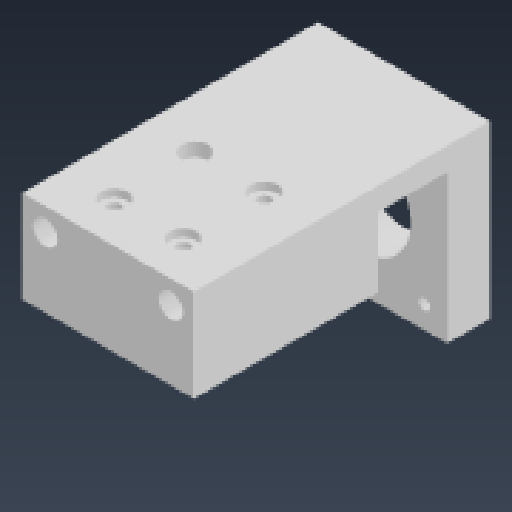
# Autodesk Inventor part: PRINTED z motor mount right
Saved by Autodesk Inventor 2024.3 (Build 283343000, 343)
## iProperties
Created: 2024-07-29
Part Number: PRINTED z motor mount right
Material: Generic
Document SubType Name: Modeling
Designer: mateu
Density: 1 g/cm^3
Appearance: Default
Author: mateu
Autodesk Inventor part; units mm, degrees
ref_plane "YZ Plane" through (0, 0, 0) normal (1, 0, 0) x (0, 1, 0)
ref_plane "XZ Plane" through (0, 0, 0) normal (0, 1, 0) x (-1, 0, 0)
ref_plane "XY Plane" through (0, 0, 0) normal (0, 0, 1) x (1, 0, 0)
sketch "Sketch1" plane through (0, 0, 0) normal (0, 0, 1) x (1, 0, 0)
  line L0 (21.025, -17.1393) -> (17.0778, -21.075) projected
  line L1 (21.075, 17.0778) -> (21.025, -17.1393) projected
  line L2 (17.1393, 21.025) -> (21.075, 17.0778) projected
  line L3 (-17.0778, 21.075) -> (17.1393, 21.025) projected
  line L4 (-21.025, 17.1393) -> (-17.0778, 21.075) projected
  line L5 (-21.075, -17.0778) -> (-21.025, 17.1393) projected
  line L6 (-17.1393, -21.025) -> (-21.075, -17.0778) projected
  line L7 (17.0778, -21.075) -> (-17.1393, -21.025) projected
  circle A0 centre (-15.5226, -15.4774) radius 1.3645 projected
  circle A1 centre (15.5226, 15.4774) radius 1.3645 projected
  circle A2 centre (0, 0) radius 11.1 projected
  circle A3 centre (-15.4774, 15.5226) radius 1.3645 projected
  circle A4 centre (15.4774, -15.5226) radius 1.3645 projected
  circle A5 centre (0, 0) radius 12.1
  line L8 (21.075, 17.0778) -> (17.1393, 17.0778)
  line L9 (17.1393, 17.0778) -> (17.1393, 21.025)
  line L10 (17.1393, 21.025) -> (21.075, 21.025)
  line L11 (21.075, 21.025) -> (21.075, 17.0778)
  line L12 (-17.1393, -21.025) -> (-21.075, -21.025)
  line L13 (-21.075, -21.025) -> (-21.075, -17.0778)
  line L14 (-21.075, -17.0778) -> (-17.1393, -17.0778)
  line L15 (-17.1393, -17.0778) -> (-17.1393, -21.025)
  line L16 (-17.1394, -21.125) -> (17.0777, -21.175) projected
  line L17 (-21.125, 17.1394) -> (-21.175, -17.0777) projected
  line L18 (21.125, -17.1394) -> (21.175, 17.0777) projected
  line L19 (17.1394, 21.125) -> (-17.0777, 21.175) projected
  line L20 (17.1394, 21.125) -> (21.175, 21.125)
  line L21 (21.175, 21.125) -> (21.175, 17.0777)
  line L22 (21.175, 17.0777) -> (17.1394, 17.0777)
  line L23 (17.1394, 17.0777) -> (17.1394, 21.125)
  line L24 (-17.1394, -21.125) -> (-21.175, -21.125)
  line L25 (-21.175, -21.125) -> (-21.175, -17.0777)
  line L26 (-21.175, -17.0777) -> (-17.1394, -17.0777)
  line L27 (-17.1394, -17.0777) -> (-17.1394, -21.125)
  line L28 (-21.175, -21.125) -> (21.175, -21.125)
  line L29 (21.175, -21.125) -> (21.175, 21.125)
  line L30 (21.175, 21.125) -> (-21.175, 21.125)
  line L31 (-21.175, 21.125) -> (-21.175, -21.125)
  point P0 (0, 0)
  dimension "d0" = 1
  constraints: 40 end point, 10 parallel, 5 horizontal, 5 perpendicular, 1 centre point
  measures "d0" radial gap between concentric circles of A2 A5
extrude "Extrusion1" add sketch "Sketch1" along normal blind 7.5 contours L1 L22 L29 L28 L27 L7 L0 | L0 L7 L15 L14 L5 L4 L3 L9 L8 L1 | L8 L9 L2 | L2 L10 L11 | L11 L10 L23 L20 L21 L22 | L12 L13 L6 | L27 L24 L25 L26 L13 L12 | L6 L14 L15 | L3 L4 L5 L26 L31 L30 L23
sketch "Sketch2" plane through (0, 0, 7.5) normal (0, 0, 1) x (1, 0, 0)
  arc A0 (-1.3547, 7.0848) -> (-1.824, -6.9788) centre (0, 0) ccw
  line L0 (-1.824, -6.9788) -> (52.9102, -21.2846)
  arc A1 (52.9102, -21.2846) -> (54.2116, 17.7095) centre (57.9677, -1.9346) ccw
  line L1 (54.2116, 17.7095) -> (-1.3547, 7.0848)
  line L2 (1.9235, 5.7586) -> (49.8414, 14.9208)
  arc A2 (50.6727, 15.052) -> (49.8414, 14.9208) centre (50.2992, 14.7197) ccw
  line L3 (50.6727, 15.052) -> (50.6801, 15.0435)
  spline S0 degree 3 poles (50.6801, 15.0435) (50.7219, 14.9959) (50.7686, 14.9492) (50.8593, 14.8771) (50.9053, 14.847) (50.9855, 14.8139) (51.0188, 14.8048) (51.0975, 14.7994) (51.1299, 14.8087) (51.1978, 14.8319) (51.2575, 14.8594) (51.2738, 14.8659) knots 0 0 0 0 0.221578 0.221578 0.405224 0.405224 0.524808 0.524808 0.681199 0.681199 1 1 1 1
  spline S1 degree 3 poles (51.2738, 14.8659) (51.3213, 14.8848) (51.3717, 14.8983) (51.4381, 14.9355) (51.4654, 14.9544) (51.5177, 15.0213) (51.536, 15.06) (51.5803, 15.1932) (51.5866, 15.3045) (51.5828, 15.4032) knots 0 0 0 0 0.321396 0.321396 0.48066 0.48066 0.635294 0.635294 1 1 1 1
  line L4 (51.5828, 15.4032) -> (51.5823, 15.4144)
  arc A3 (52.4883, 15.7215) -> (51.5823, 15.4144) centre (52.082, 15.43) ccw
  ellipse E0 centre (52.6181, 16.5825) end of major axis (52.9222, 15.4382) minor radius 0.4695 (52.4883, 15.7215) -> (52.7342, 15.4739) ccw
  line L5 (52.7342, 15.4739) -> (53.3062, 15.5833)
  spline S2 degree 3 poles (53.3062, 15.5833) (53.3285, 15.6089) (53.3465, 15.6383) (53.3759, 15.7001) (53.3876, 15.7332) (53.4154, 15.8335) (53.4254, 15.9062) (53.43, 15.9756) knots 0 0 0 0 0.246113 0.246113 0.495831 0.495831 1 1 1 1
  line L6 (53.43, 15.9756) -> (53.4307, 15.9869)
  arc A4 (54.3639, 16.1976) -> (53.4307, 15.9869) centre (53.9294, 15.9501) ccw
  line L7 (54.3639, 16.1976) -> (54.3693, 16.1877)
  spline S3 degree 3 poles (54.3693, 16.1877) (54.4048, 16.1244) (54.4473, 16.0602) (54.5277, 15.9698) (54.5647, 15.9356) (54.6338, 15.8924) (54.664, 15.8787) (54.7363, 15.8619) (54.7701, 15.8644) (54.8153, 15.8718) knots 0 0 0 0 0.371919 0.371919 0.619946 0.619946 0.788977 0.788977 1 1 1 1
  line L8 (54.8153, 15.8718) -> (54.9027, 15.8885)
  spline S4 degree 3 poles (54.9027, 15.8885) (54.9046, 15.8889) (54.9067, 15.8893) (54.91, 15.89) (54.9117, 15.8903) (54.9132, 15.8905) knots 0 0 0 0 0.573872 0.573872 1 1 1 1
  line L9 (54.9132, 15.8905) -> (55.0804, 15.9225)
  spline S5 degree 3 poles (55.0804, 15.9225) (55.0932, 15.9274) (55.1129, 15.936) (55.1525, 15.9644) (55.1681, 15.9786) (55.2105, 16.0255) (55.2333, 16.0625) (55.2889, 16.1774) (55.3125, 16.2676) (55.327, 16.3518) knots 0 0 0 0 0.157005 0.157005 0.276336 0.276336 0.51523 0.51523 1 1 1 1
  line L10 (55.327, 16.3518) -> (55.3289, 16.3629)
  arc A5 (56.2789, 16.4749) -> (55.3289, 16.3629) centre (55.821, 16.2743) ccw
  ellipse E1 centre (56.5798, 17.2686) end of major axis (56.6442, 16.1081) minor radius 0.4625 (56.2789, 16.4749) -> (56.4624, 16.1868) ccw
  line L11 (56.4624, 16.1868) -> (57.173, 16.3227)
  ellipse E2 centre (56.96, 17.031) end of major axis (56.9523, 16.1396) minor radius 0.3594 (57.173, 16.3227) -> (57.2529, 16.5276) ccw
  line L12 (57.2529, 16.5276) -> (57.256, 16.5385)
  arc A6 (58.2125, 16.5506) -> (57.256, 16.5385) centre (57.7361, 16.3989) ccw
  line L13 (58.2125, 16.5506) -> (58.2158, 16.5398)
  ellipse E3 centre (58.3562, 16.7592) end of major axis (58.4541, 16.2126) minor radius 0.1884 (58.2158, 16.5398) -> (58.2211, 16.5231) ccw
  line L14 (58.2211, 16.5231) -> (59.3878, 16.7461)
  arc A7 (60.1434, 16.4238) -> (59.3878, 16.7461) centre (59.6537, 16.3227) ccw
  line L15 (60.1434, 16.4238) -> (60.1456, 16.4127)
  spline S6 degree 3 poles (60.1456, 16.4127) (60.1579, 16.3506) (60.175, 16.2867) (60.2175, 16.1789) (60.2423, 16.1299) (60.2952, 16.0611) (60.3195, 16.0366) (60.385, 15.9926) (60.4177, 15.9844) (60.4881, 15.9705) (60.5536, 15.9645) (60.5709, 15.962) knots 0 0 0 0 0.221578 0.221578 0.405224 0.405224 0.524808 0.524808 0.681199 0.681199 1 1 1 1
  spline S7 degree 3 poles (60.5709, 15.962) (60.6214, 15.9546) (60.6719, 15.9411) (60.7479, 15.9402) (60.7811, 15.9429) (60.8598, 15.9747) (60.895, 15.999) (61, 16.0922) (61.0611, 16.1855) (61.1071, 16.2728) knots 0 0 0 0 0.321396 0.321396 0.48066 0.48066 0.635294 0.635294 1 1 1 1
  line L16 (61.1071, 16.2728) -> (61.1123, 16.2828)
  arc A8 (62.0505, 16.0958) -> (61.1123, 16.2828) centre (61.5529, 16.0464) ccw
  line L17 (62.0505, 16.0958) -> (62.0514, 16.0845)
  spline S8 degree 3 poles (62.0514, 16.0845) (62.0572, 16.0215) (62.0676, 15.9562) (62.0985, 15.8445) (62.1181, 15.7932) (62.1635, 15.7193) (62.1851, 15.6924) (62.2456, 15.6417) (62.2773, 15.6302) (62.3459, 15.609) (62.4104, 15.5962) (62.4274, 15.5919) knots 0 0 0 0 0.221578 0.221578 0.405224 0.405224 0.524808 0.524808 0.681199 0.681199 1 1 1 1
  spline S9 degree 3 poles (62.4274, 15.5919) (62.4768, 15.5792) (62.5256, 15.5605) (62.6011, 15.5516) (62.6344, 15.5509) (62.716, 15.5743) (62.7536, 15.5948) (62.8677, 15.6765) (62.9382, 15.7629) (62.9931, 15.8449) knots 0 0 0 0 0.321396 0.321396 0.48066 0.48066 0.635294 0.635294 1 1 1 1
  line L18 (62.9931, 15.8449) -> (62.9993, 15.8543)
  arc A9 (63.9128, 15.5702) -> (62.9993, 15.8543) centre (63.4128, 15.5732) ccw
  line L19 (63.9128, 15.5702) -> (63.9126, 15.5589)
  spline S10 degree 3 poles (63.9126, 15.5589) (63.9118, 15.4956) (63.9152, 15.4296) (63.9343, 15.3154) (63.9484, 15.2622) (63.9858, 15.184) (64.0045, 15.155) (64.0594, 15.0982) (64.0897, 15.0835) (64.1557, 15.0553) (64.2185, 15.0358) (64.235, 15.0297) knots 0 0 0 0 0.221578 0.221578 0.405224 0.405224 0.524808 0.524808 0.681199 0.681199 1 1 1 1
  spline S11 degree 3 poles (64.235, 15.0297) (64.2828, 15.012) (64.3294, 14.9883) (64.4035, 14.9715) (64.4366, 14.9673) (64.5201, 14.982) (64.5597, 14.9985) (64.6817, 15.0679) (64.7608, 15.1464) (64.824, 15.2222) knots 0 0 0 0 0.321396 0.321396 0.48066 0.48066 0.635294 0.635294 1 1 1 1
  line L20 (64.824, 15.2222) -> (64.8312, 15.2309)
  arc A10 (65.71, 14.8529) -> (64.8312, 15.2309) centre (65.213, 14.9081) ccw
  line L21 (65.71, 14.8529) -> (65.7086, 14.8417)
  spline S12 degree 3 poles (65.7086, 14.8417) (65.7012, 14.7788) (65.6977, 14.7128) (65.7048, 14.5972) (65.7132, 14.5428) (65.7423, 14.4611) (65.7578, 14.4303) (65.8065, 14.3682) (65.8351, 14.3503) (65.8977, 14.3154) (65.9581, 14.2894) (65.9739, 14.2817) knots 0 0 0 0 0.221578 0.221578 0.405224 0.405224 0.524808 0.524808 0.681199 0.681199 1 1 1 1
  spline S13 degree 3 poles (65.9739, 14.2817) (66.0196, 14.259) (66.0634, 14.2306) (66.1355, 14.2062) (66.1679, 14.1985) (66.2525, 14.2044) (66.2935, 14.2167) (66.4222, 14.2729) (66.5091, 14.3428) (66.5798, 14.4116) knots 0 0 0 0 0.321396 0.321396 0.48066 0.48066 0.635294 0.635294 1 1 1 1
  line L22 (66.5798, 14.4116) -> (66.5879, 14.4195)
  arc A11 (67.4223, 13.9517) -> (66.5879, 14.4195) centre (66.9339, 14.0585) ccw
  line L23 (67.4223, 13.9517) -> (67.4198, 13.9407)
  spline S14 degree 3 poles (67.4198, 13.9407) (67.4058, 13.8789) (67.3955, 13.8136) (67.3904, 13.6979) (67.3932, 13.643) (67.4135, 13.5587) (67.4257, 13.5264) (67.4676, 13.4595) (67.4942, 13.4388) (67.5529, 13.3974) (67.6102, 13.3653) (67.6251, 13.356) knots 0 0 0 0 0.221578 0.221578 0.405224 0.405224 0.524808 0.524808 0.681199 0.681199 1 1 1 1
  spline S15 degree 3 poles (67.6251, 13.356) (67.6682, 13.3287) (67.7088, 13.2958) (67.7779, 13.264) (67.8093, 13.253) (67.8941, 13.25) (67.9362, 13.2579) (68.07, 13.3004) (68.1637, 13.3608) (68.2413, 13.4218) knots 0 0 0 0 0.321396 0.321396 0.48066 0.48066 0.635294 0.635294 1 1 1 1
  line L24 (68.2413, 13.4218) -> (68.2501, 13.4288)
  arc A12 (69.0311, 12.8764) -> (68.2501, 13.4288) centre (68.5565, 13.0337) ccw
  line L25 (69.0311, 12.8764) -> (69.0274, 12.8657)
  spline S16 degree 3 poles (69.0274, 12.8657) (69.0071, 12.8057) (68.99, 12.7419) (68.9729, 12.6273) (68.9698, 12.5724) (68.9812, 12.4864) (68.9901, 12.4531) (69.0247, 12.3822) (69.049, 12.3588) (69.103, 12.3115) (69.1567, 12.2736) (69.1705, 12.2627) knots 0 0 0 0 0.221578 0.221578 0.405224 0.405224 0.524808 0.524808 0.681199 0.681199 1 1 1 1
  spline S17 degree 3 poles (69.1705, 12.2627) (69.2105, 12.2311) (69.2475, 12.1941) (69.3128, 12.1553) (69.3429, 12.1411) (69.427, 12.1293) (69.4696, 12.1327) (69.6072, 12.161) (69.7067, 12.2112) (69.7902, 12.2638) knots 0 0 0 0 0.321396 0.321396 0.48066 0.48066 0.635294 0.635294 1 1 1 1
  line L26 (69.7902, 12.2638) -> (69.7997, 12.2699)
  arc A13 (70.5187, 11.6388) -> (69.7997, 12.2699) centre (70.0631, 11.8448) ccw
  line L27 (70.5187, 11.6388) -> (70.5139, 11.6285)
  spline S18 degree 3 poles (70.5139, 11.6285) (70.4874, 11.571) (70.4637, 11.5093) (70.4347, 11.3972) (70.426, 11.3429) (70.4283, 11.2562) (70.4336, 11.2221) (70.4607, 11.148) (70.4824, 11.1221) (70.5311, 11.0695) (70.5806, 11.0262) (70.5932, 11.0139) knots 0 0 0 0 0.221578 0.221578 0.405224 0.405224 0.524808 0.524808 0.681199 0.681199 1 1 1 1
  spline S19 degree 3 poles (70.5932, 11.0139) (70.6297, 10.9783) (70.6625, 10.9377) (70.7235, 10.8922) (70.7519, 10.8749) (70.8343, 10.8544) (70.8771, 10.8533) (71.0168, 10.8671) (71.121, 10.9067) (71.2096, 10.9502) knots 0 0 0 0 0.321396 0.321396 0.48066 0.48066 0.635294 0.635294 1 1 1 1
  line L28 (71.2096, 10.9502) -> (71.2197, 10.9553)
  arc A14 (71.8687, 10.2525) -> (71.2197, 10.9553) centre (71.4372, 10.5051) ccw
  line L29 (71.8687, 10.2525) -> (71.8629, 10.2428)
  spline S20 degree 3 poles (71.8629, 10.2428) (71.8305, 10.1884) (71.8005, 10.1295) (71.76, 10.021) (71.7456, 9.9679) (71.7389, 9.8815) (71.7406, 9.847) (71.7597, 9.7704) (71.7786, 9.7425) (71.8216, 9.6851) (71.8663, 9.6368) (71.8775, 9.6233) knots 0 0 0 0 0.221578 0.221578 0.405224 0.405224 0.524808 0.524808 0.681199 0.681199 1 1 1 1
  spline S21 degree 3 poles (71.8775, 9.6233) (71.9101, 9.584) (71.9385, 9.5402) (71.9944, 9.4886) (72.0209, 9.4684) (72.1006, 9.4394) (72.1431, 9.4339) (72.2835, 9.433) (72.3913, 9.4614) (72.4839, 9.4955) knots 0 0 0 0 0.321396 0.321396 0.48066 0.48066 0.635294 0.635294 1 1 1 1
  line L30 (72.4839, 9.4955) -> (72.4945, 9.4994)
  arc A15 (73.0665, 8.7327) -> (72.4945, 9.4994) centre (72.6637, 9.029) ccw
  line L31 (73.0665, 8.7327) -> (73.0597, 8.7237)
  spline S22 degree 3 poles (73.0597, 8.7237) (73.0218, 8.6729) (72.9858, 8.6175) (72.9341, 8.5138) (72.9143, 8.4625) (72.8986, 8.3773) (72.8966, 8.3428) (72.9077, 8.2646) (72.9235, 8.2349) (72.9603, 8.1733) (72.9997, 8.1206) (73.0094, 8.106) knots 0 0 0 0 0.221578 0.221578 0.405224 0.405224 0.524808 0.524808 0.681199 0.681199 1 1 1 1
  spline S23 degree 3 poles (73.0094, 8.106) (73.0377, 8.0635) (73.0614, 8.017) (73.1116, 7.9598) (73.1358, 7.937) (73.2121, 7.8998) (73.2537, 7.8899) (73.3933, 7.8743) (73.5035, 7.8913) (73.5991, 7.9155) knots 0 0 0 0 0.321396 0.321396 0.48066 0.48066 0.635294 0.635294 1 1 1 1
  line L32 (73.5991, 7.9155) -> (73.6101, 7.9184)
  arc A16 (74.0988, 7.096) -> (73.6101, 7.9184) centre (73.7292, 7.4328) ccw
  line L33 (74.0988, 7.096) -> (74.0911, 7.0877)
  spline S24 degree 3 poles (74.0911, 7.0877) (74.0538, 7.0474) (74.0178, 7.0036) (73.9564, 6.9135) (73.9287, 6.8641) (73.899, 6.7792) (73.8911, 6.7436) (73.8895, 6.6778) (73.8937, 6.6486) (73.9222, 6.5681) (73.9723, 6.4867) (74.0009, 6.4323) knots 0 0 0 0 0.238639 0.238639 0.473417 0.473417 0.629303 0.629303 0.759091 0.759091 1 1 1 1
  spline S25 degree 3 poles (74.0009, 6.4323) (74.0244, 6.387) (74.043, 6.3382) (74.0868, 6.276) (74.1084, 6.2507) (74.1802, 6.2055) (74.2206, 6.1912) (74.3576, 6.1607) (74.469, 6.1658) (74.5667, 6.1796) knots 0 0 0 0 0.321396 0.321396 0.48066 0.48066 0.635294 0.635294 1 1 1 1
  line L34 (74.5667, 6.1796) -> (74.5779, 6.1812)
  arc A17 (74.9755, 5.3111) -> (74.5779, 6.1812) centre (74.6442, 5.6856) ccw
  line L35 (74.9755, 5.3111) -> (74.9669, 5.3037)
  spline S26 degree 3 poles (74.9669, 5.3037) (74.9192, 5.2621) (74.8723, 5.2155) (74.7999, 5.125) (74.7697, 5.0791) (74.7364, 4.999) (74.7273, 4.9658) (74.7216, 4.887) (74.7308, 4.8546) (74.7538, 4.7866) (74.7812, 4.7269) (74.7876, 4.7105) knots 0 0 0 0 0.221578 0.221578 0.405224 0.405224 0.524808 0.524808 0.681199 0.681199 1 1 1 1
  spline S27 degree 3 poles (74.7876, 4.7105) (74.8063, 4.663) (74.8197, 4.6126) (74.8567, 4.5461) (74.8756, 4.5187) (74.9423, 4.4662) (74.9809, 4.4478) (75.114, 4.4031) (75.2253, 4.3965) (75.3239, 4.4) knots 0 0 0 0 0.321396 0.321396 0.48066 0.48066 0.635294 0.635294 1 1 1 1
  line L36 (75.3239, 4.4) -> (75.3352, 4.4005)
  arc A18 (75.6397, 3.4936) -> (75.3352, 4.4005) centre (75.3494, 3.9007) ccw
  line L37 (75.6397, 3.4936) -> (75.6304, 3.4872)
  spline S28 degree 3 poles (75.6304, 3.4872) (75.5786, 3.4508) (75.5271, 3.4093) (75.4457, 3.3269) (75.4108, 3.2844) (75.3693, 3.2083) (75.3567, 3.1761) (75.3429, 3.0984) (75.3487, 3.0652) (75.3644, 2.9952) (75.3854, 2.9329) (75.3901, 2.916) knots 0 0 0 0 0.221578 0.221578 0.405224 0.405224 0.524808 0.524808 0.681199 0.681199 1 1 1 1
  spline S29 degree 3 poles (75.3901, 2.916) (75.4037, 2.8668) (75.4118, 2.8152) (75.4416, 2.7452) (75.4575, 2.716) (75.5184, 2.6569) (75.5549, 2.6344) (75.6826, 2.5761) (75.7926, 2.5579) (75.891, 2.5511) knots 0 0 0 0 0.321396 0.321396 0.48066 0.48066 0.635294 0.635294 1 1 1 1
  line L38 (75.891, 2.5511) -> (75.9023, 2.5504)
  arc A19 (76.1103, 1.6167) -> (75.9023, 2.5504) centre (75.8641, 2.0518) ccw
  line L39 (76.1103, 1.6167) -> (76.1004, 1.6112)
  spline S30 degree 3 poles (76.1004, 1.6112) (76.045, 1.5804) (75.9895, 1.5446) (75.8999, 1.4711) (75.8608, 1.4325) (75.8116, 1.3611) (75.7957, 1.3305) (75.7738, 1.2546) (75.7761, 1.221) (75.7844, 1.1497) (75.7987, 1.0856) (75.8017, 1.0683) knots 0 0 0 0 0.221578 0.221578 0.405224 0.405224 0.524808 0.524808 0.681199 0.681199 1 1 1 1
  spline S31 degree 3 poles (75.8017, 1.0683) (75.8101, 1.0179) (75.8127, 0.9658) (75.8351, 0.8931) (75.8478, 0.8623) (75.9022, 0.7972) (75.9361, 0.7711) (76.057, 0.6997) (76.1645, 0.6701) (76.2617, 0.6531) knots 0 0 0 0 0.321396 0.321396 0.48066 0.48066 0.635294 0.635294 1 1 1 1
  line L40 (76.2617, 0.6531) -> (76.2729, 0.6511)
  arc A20 (76.3821, -0.2992) -> (76.2729, 0.6511) centre (76.1828, 0.1593) ccw
  line L41 (76.3821, -0.2992) -> (76.3717, -0.3036)
  spline S32 degree 3 poles (76.3717, -0.3036) (76.3134, -0.3284) (76.2545, -0.3583) (76.1577, -0.4219) (76.1147, -0.4563) (76.0583, -0.5221) (76.0393, -0.551) (76.0096, -0.6241) (76.0084, -0.6578) (76.0092, -0.7295) (76.0168, -0.7948) (76.0179, -0.8124) knots 0 0 0 0 0.221578 0.221578 0.405224 0.405224 0.524808 0.524808 0.681199 0.681199 1 1 1 1
  spline S33 degree 3 poles (76.0179, -0.8124) (76.021, -0.8633) (76.0181, -0.9154) (76.0327, -0.9901) (76.0422, -1.022) (76.0895, -1.0925) (76.1205, -1.122) (76.2333, -1.2056) (76.3371, -1.2462) (76.432, -1.2734) knots 0 0 0 0 0.321396 0.321396 0.48066 0.48066 0.635294 0.635294 1 1 1 1
  line L42 (76.432, -1.2734) -> (76.4429, -1.2764)
  arc A21 (76.4522, -2.233) -> (76.4429, -1.2764) centre (76.3019, -1.7561) ccw
  line L43 (76.4522, -2.233) -> (76.4414, -2.2363)
  spline S34 degree 3 poles (76.4414, -2.2363) (76.3627, -2.2604) (76.2801, -2.2935) (76.1728, -2.3609) (76.1366, -2.3891) (76.0864, -2.4465) (76.069, -2.4732) (76.0327, -2.5639) (76.0404, -2.6175) (76.0375, -2.6791) knots 0 0 0 0 0.366803 0.366803 0.564574 0.564574 0.706452 0.706452 1 1 1 1
  spline S35 degree 3 poles (76.0375, -2.6791) (76.0361, -2.7187) (76.0306, -2.7591) (76.0338, -2.8213) (76.0381, -2.8537) (76.075, -2.9302) (76.102, -2.9635) (76.206, -3.0625) (76.3091, -3.1158) (76.4036, -3.1536) knots 0 0 0 0 0.287377 0.287377 0.45164 0.45164 0.61189 0.61189 1 1 1 1
  line L44 (76.4036, -3.1536) -> (76.4141, -3.1577)
  arc A22 (76.3261, -4.1103) -> (76.4141, -3.1577) centre (76.225, -3.6206) ccw
  line L45 (76.3261, -4.1103) -> (76.315, -4.1125)
  spline S36 degree 3 poles (76.315, -4.1125) (76.2529, -4.1248) (76.1891, -4.1419) (76.0813, -4.1844) (76.0322, -4.2092) (75.9635, -4.2621) (75.939, -4.2864) (75.8949, -4.3519) (75.8868, -4.3846) (75.8729, -4.455) (75.8669, -4.5205) (75.8644, -4.5378) knots 0 0 0 0 0.221578 0.221578 0.405224 0.405224 0.524808 0.524808 0.681199 0.681199 1 1 1 1
  spline S37 degree 3 poles (75.8644, -4.5378) (75.857, -4.5883) (75.8435, -4.6388) (75.8425, -4.7148) (75.8452, -4.748) (75.877, -4.8267) (75.9013, -4.8619) (75.9946, -4.9669) (76.0879, -5.028) (76.1752, -5.074) knots 0 0 0 0 0.321396 0.321396 0.48066 0.48066 0.635294 0.635294 1 1 1 1
  line L46 (76.1752, -5.074) -> (76.1852, -5.0792)
  arc A23 (75.9981, -6.0174) -> (76.1852, -5.0792) centre (75.9488, -5.5198) ccw
  line L47 (75.9981, -6.0174) -> (75.9869, -6.0183)
  spline S38 degree 3 poles (75.9869, -6.0183) (75.9238, -6.0241) (75.8585, -6.0345) (75.7469, -6.0654) (75.6955, -6.085) (75.6216, -6.1304) (75.5947, -6.152) (75.544, -6.2125) (75.5325, -6.2442) (75.5114, -6.3128) (75.4985, -6.3773) (75.4942, -6.3943) knots 0 0 0 0 0.221578 0.221578 0.405224 0.405224 0.524808 0.524808 0.681199 0.681199 1 1 1 1
  spline S39 degree 3 poles (75.4942, -6.3943) (75.4816, -6.4437) (75.4629, -6.4925) (75.454, -6.568) (75.4532, -6.6013) (75.4766, -6.6829) (75.4971, -6.7205) (75.5789, -6.8346) (75.6653, -6.9051) (75.7473, -6.96) knots 0 0 0 0 0.321396 0.321396 0.48066 0.48066 0.635294 0.635294 1 1 1 1
  line L48 (75.7473, -6.96) -> (75.7567, -6.9662)
  arc A24 (75.4726, -7.8797) -> (75.7567, -6.9662) centre (75.4755, -7.3797) ccw
  line L49 (75.4726, -7.8797) -> (75.4613, -7.8795)
  spline S40 degree 3 poles (75.4613, -7.8795) (75.398, -7.8787) (75.332, -7.8821) (75.2177, -7.9012) (75.1646, -7.9153) (75.0863, -7.9527) (75.0573, -7.9714) (75.0006, -8.0263) (74.9858, -8.0566) (74.9576, -8.1226) (74.9381, -8.1854) (74.9321, -8.2019) knots 0 0 0 0 0.221578 0.221578 0.405224 0.405224 0.524808 0.524808 0.681199 0.681199 1 1 1 1
  spline S41 degree 3 poles (74.9321, -8.2019) (74.9143, -8.2497) (74.8906, -8.2963) (74.8739, -8.3704) (74.8696, -8.4035) (74.8844, -8.487) (74.9008, -8.5266) (74.9702, -8.6486) (75.0488, -8.7277) (75.1246, -8.7909) knots 0 0 0 0 0.321396 0.321396 0.48066 0.48066 0.635294 0.635294 1 1 1 1
  line L50 (75.1246, -8.7909) -> (75.1333, -8.7981)
  arc A25 (74.7553, -9.6769) -> (75.1333, -8.7981) centre (74.8105, -9.1799) ccw
  line L51 (74.7553, -9.6769) -> (74.7441, -9.6755)
  spline S42 degree 3 poles (74.7441, -9.6755) (74.6812, -9.6681) (74.6152, -9.6646) (74.4995, -9.6717) (74.4452, -9.6801) (74.3635, -9.7092) (74.3327, -9.7247) (74.2705, -9.7734) (74.2527, -9.802) (74.2177, -9.8646) (74.1918, -9.925) (74.184, -9.9408) knots 0 0 0 0 0.221578 0.221578 0.405224 0.405224 0.524808 0.524808 0.681199 0.681199 1 1 1 1
  spline S43 degree 3 poles (74.184, -9.9408) (74.1614, -9.9865) (74.1329, -10.0303) (74.1085, -10.1024) (74.1009, -10.1348) (74.1068, -10.2194) (74.119, -10.2604) (74.1753, -10.3891) (74.2451, -10.476) (74.3139, -10.5467) knots 0 0 0 0 0.321396 0.321396 0.48066 0.48066 0.635294 0.635294 1 1 1 1
  line L52 (74.3139, -10.5467) -> (74.3218, -10.5548)
  arc A26 (73.854, -11.3892) -> (74.3218, -10.5548) centre (73.9609, -10.9008) ccw
  line L53 (73.854, -11.3892) -> (73.843, -11.3867)
  spline S44 degree 3 poles (73.843, -11.3867) (73.7812, -11.3727) (73.716, -11.3624) (73.6002, -11.3573) (73.5453, -11.3601) (73.461, -11.3804) (73.4287, -11.3926) (73.3618, -11.4345) (73.3411, -11.4611) (73.2998, -11.5198) (73.2677, -11.5771) (73.2583, -11.592) knots 0 0 0 0 0.221578 0.221578 0.405224 0.405224 0.524808 0.524808 0.681199 0.681199 1 1 1 1
  spline S45 degree 3 poles (73.2583, -11.592) (73.231, -11.6351) (73.1982, -11.6757) (73.1663, -11.7448) (73.1553, -11.7762) (73.1524, -11.861) (73.1603, -11.9031) (73.2028, -12.0369) (73.2631, -12.1306) (73.3242, -12.2082) knots 0 0 0 0 0.321396 0.321396 0.48066 0.48066 0.635294 0.635294 1 1 1 1
  line L54 (73.3242, -12.2082) -> (73.3312, -12.217)
  arc A27 (72.7787, -12.998) -> (73.3312, -12.217) centre (72.936, -12.5234) ccw
  line L55 (72.7787, -12.998) -> (72.768, -12.9943)
  spline S46 degree 3 poles (72.768, -12.9943) (72.7081, -12.974) (72.6442, -12.9569) (72.5296, -12.9398) (72.4747, -12.9367) (72.3888, -12.9481) (72.3554, -12.957) (72.2845, -12.9916) (72.2611, -13.0159) (72.2139, -13.0699) (72.1759, -13.1236) (72.1651, -13.1374) knots 0 0 0 0 0.221578 0.221578 0.405224 0.405224 0.524808 0.524808 0.681199 0.681199 1 1 1 1
  spline S47 degree 3 poles (72.1651, -13.1374) (72.1334, -13.1774) (72.0965, -13.2144) (72.0576, -13.2797) (72.0434, -13.3098) (72.0316, -13.3939) (72.035, -13.4365) (72.0633, -13.5741) (72.1136, -13.6736) (72.1662, -13.7571) knots 0 0 0 0 0.321396 0.321396 0.48066 0.48066 0.635294 0.635294 1 1 1 1
  line L56 (72.1662, -13.7571) -> (72.1722, -13.7666)
  arc A28 (71.5411, -14.4856) -> (72.1722, -13.7666) centre (71.7472, -14.03) ccw
  line L57 (71.5411, -14.4856) -> (71.5309, -14.4808)
  spline S48 degree 3 poles (71.5309, -14.4808) (71.4734, -14.4543) (71.4117, -14.4306) (71.2995, -14.4016) (71.2452, -14.3929) (71.1586, -14.3952) (71.1244, -14.4005) (71.0503, -14.4276) (71.0245, -14.4493) (70.9719, -14.498) (70.9285, -14.5475) (70.9163, -14.5601) knots 0 0 0 0 0.221578 0.221578 0.405224 0.405224 0.524808 0.524808 0.681199 0.681199 1 1 1 1
  spline S49 degree 3 poles (70.9163, -14.5601) (70.8806, -14.5966) (70.84, -14.6294) (70.7946, -14.6904) (70.7773, -14.7188) (70.7567, -14.8012) (70.7557, -14.844) (70.7695, -14.9837) (70.809, -15.0879) (70.8526, -15.1765) knots 0 0 0 0 0.321396 0.321396 0.48066 0.48066 0.635294 0.635294 1 1 1 1
  line L58 (70.8526, -15.1765) -> (70.8576, -15.1866)
  arc A29 (70.1549, -15.8356) -> (70.8576, -15.1866) centre (70.4074, -15.4041) ccw
  line L59 (70.1549, -15.8356) -> (70.1452, -15.8298)
  spline S50 degree 3 poles (70.1452, -15.8298) (70.0907, -15.7974) (70.0319, -15.7674) (69.9233, -15.7269) (69.8703, -15.7125) (69.7838, -15.7058) (69.7493, -15.7075) (69.6728, -15.7266) (69.6448, -15.7455) (69.5874, -15.7885) (69.5391, -15.8332) (69.5256, -15.8444) knots 0 0 0 0 0.221578 0.221578 0.405224 0.405224 0.524808 0.524808 0.681199 0.681199 1 1 1 1
  spline S51 degree 3 poles (69.5256, -15.8444) (69.4864, -15.877) (69.4426, -15.9054) (69.391, -15.9613) (69.3708, -15.9878) (69.3418, -16.0675) (69.3362, -16.11) (69.3353, -16.2503) (69.3638, -16.3582) (69.3979, -16.4508) knots 0 0 0 0 0.321396 0.321396 0.48066 0.48066 0.635294 0.635294 1 1 1 1
  line L60 (69.3979, -16.4508) -> (69.4018, -16.4614)
  arc A30 (68.635, -17.0334) -> (69.4018, -16.4614) centre (68.9313, -16.6306) ccw
  line L61 (68.635, -17.0334) -> (68.626, -17.0266)
  spline S52 degree 3 poles (68.626, -17.0266) (68.5753, -16.9887) (68.5198, -16.9527) (68.4162, -16.901) (68.3649, -16.8812) (68.2796, -16.8655) (68.2451, -16.8635) (68.167, -16.8746) (68.1372, -16.8904) (68.0756, -16.9272) (68.023, -16.9666) (68.0084, -16.9763) knots 0 0 0 0 0.221578 0.221578 0.405224 0.405224 0.524808 0.524808 0.681199 0.681199 1 1 1 1
  spline S53 degree 3 poles (68.0084, -16.9763) (67.9659, -17.0046) (67.9194, -17.0283) (67.8622, -17.0785) (67.8394, -17.1027) (67.8022, -17.179) (67.7922, -17.2206) (67.7767, -17.3602) (67.7937, -17.4704) (67.8179, -17.566) knots 0 0 0 0 0.321396 0.321396 0.48066 0.48066 0.635294 0.635294 1 1 1 1
  line L62 (67.8179, -17.566) -> (67.8207, -17.577)
  arc A31 (66.9984, -18.0657) -> (67.8207, -17.577) centre (67.3351, -17.6961) ccw
  line L63 (66.9984, -18.0657) -> (66.9901, -18.058)
  spline S54 degree 3 poles (66.9901, -18.058) (66.9436, -18.015) (66.8922, -17.9734) (66.7945, -17.9112) (66.7456, -17.8861) (66.6624, -17.8615) (66.6283, -17.856) (66.5495, -17.8589) (66.5182, -17.8715) (66.4531, -17.9016) (66.3966, -17.9353) (66.3811, -17.9435) knots 0 0 0 0 0.221578 0.221578 0.405224 0.405224 0.524808 0.524808 0.681199 0.681199 1 1 1 1
  spline S55 degree 3 poles (66.3811, -17.9435) (66.3359, -17.9671) (66.2871, -17.9859) (66.225, -18.0298) (66.1998, -18.0515) (66.1548, -18.1235) (66.1406, -18.1638) (66.1105, -18.301) (66.1159, -18.4123) (66.13, -18.51) knots 0 0 0 0 0.321396 0.321396 0.48066 0.48066 0.635294 0.635294 1 1 1 1
  line L64 (66.13, -18.51) -> (66.1317, -18.5212)
  arc A32 (65.2627, -18.9213) -> (66.1317, -18.5212) centre (65.6363, -18.5889) ccw
  line L65 (65.2627, -18.9213) -> (65.2553, -18.9128)
  spline S56 degree 3 poles (65.2553, -18.9128) (65.2136, -18.8652) (65.1668, -18.8184) (65.0762, -18.7463) (65.0301, -18.7162) (64.95, -18.6831) (64.9167, -18.6741) (64.8379, -18.6687) (64.8055, -18.678) (64.7376, -18.7011) (64.6779, -18.7287) (64.6616, -18.7352) knots 0 0 0 0 0.221578 0.221578 0.405224 0.405224 0.524808 0.524808 0.681199 0.681199 1 1 1 1
  spline S57 degree 3 poles (64.6616, -18.7352) (64.6142, -18.754) (64.5637, -18.7676) (64.4974, -18.8047) (64.47, -18.8237) (64.4178, -18.8906) (64.3994, -18.9292) (64.3552, -19.0625) (64.3489, -19.1738) (64.3527, -19.2724) knots 0 0 0 0 0.321396 0.321396 0.48066 0.48066 0.635294 0.635294 1 1 1 1
  line L66 (64.3527, -19.2724) -> (64.3532, -19.2837)
  arc A33 (63.4472, -19.5908) -> (64.3532, -19.2837) centre (63.8534, -19.2993) ccw
  line L67 (63.4472, -19.5908) -> (63.4407, -19.5815)
  spline S58 degree 3 poles (63.4407, -19.5815) (63.4041, -19.5298) (63.3625, -19.4785) (63.2799, -19.3972) (63.2373, -19.3625) (63.161, -19.3212) (63.1288, -19.3087) (63.0511, -19.2951) (63.0179, -19.301) (62.948, -19.3169) (62.8857, -19.3381) (62.8688, -19.3429) knots 0 0 0 0 0.221578 0.221578 0.405224 0.405224 0.524808 0.524808 0.681199 0.681199 1 1 1 1
  spline S59 degree 3 poles (62.8688, -19.3429) (62.8197, -19.3566) (62.7681, -19.3648) (62.6982, -19.3949) (62.669, -19.4108) (62.6101, -19.4719) (62.5878, -19.5084) (62.5298, -19.6363) (62.512, -19.7464) (62.5054, -19.8448) knots 0 0 0 0 0.321396 0.321396 0.48066 0.48066 0.635294 0.635294 1 1 1 1
  line L68 (62.5054, -19.8448) -> (62.5047, -19.8561)
  arc A34 (61.5716, -20.0668) -> (62.5047, -19.8561) centre (62.0061, -19.8194) ccw
  line L69 (61.5716, -20.0668) -> (61.5661, -20.0569)
  spline S60 degree 3 poles (61.5661, -20.0569) (61.5352, -20.0017) (61.4992, -19.9463) (61.4255, -19.8569) (61.3867, -19.8179) (61.3152, -19.7688) (61.2845, -19.753) (61.2086, -19.7314) (61.175, -19.7338) (61.1037, -19.7423) (61.0396, -19.7568) (61.0223, -19.7598) knots 0 0 0 0 0.221578 0.221578 0.405224 0.405224 0.524808 0.524808 0.681199 0.681199 1 1 1 1
  spline S61 degree 3 poles (61.0223, -19.7598) (60.972, -19.7684) (60.9198, -19.7711) (60.8472, -19.7937) (60.8165, -19.8065) (60.7515, -19.8611) (60.7255, -19.8951) (60.6545, -20.0162) (60.6252, -20.1238) (60.6084, -20.221) knots 0 0 0 0 0.321396 0.321396 0.48066 0.48066 0.635294 0.635294 1 1 1 1
  line L70 (60.6084, -20.221) -> (60.6066, -20.2322)
  arc A35 (59.6565, -20.3442) -> (60.6066, -20.2322) centre (60.1145, -20.1435) ccw
  line L71 (59.6565, -20.3442) -> (59.6521, -20.3338)
  spline S62 degree 3 poles (59.6521, -20.3338) (59.6271, -20.2756) (59.5971, -20.2167) (59.5331, -20.1201) (59.4987, -20.0773) (59.4327, -20.021) (59.4038, -20.0021) (59.3306, -19.9726) (59.2969, -19.9715) (59.2252, -19.9725) (59.1599, -19.9803) (59.1423, -19.9814) knots 0 0 0 0 0.221578 0.221578 0.405224 0.405224 0.524808 0.524808 0.681199 0.681199 1 1 1 1
  spline S63 degree 3 poles (59.1423, -19.9814) (59.0914, -19.9847) (59.0392, -19.982) (58.9647, -19.9968) (58.9328, -20.0064) (58.8624, -20.0539) (58.833, -20.085) (58.7497, -20.198) (58.7094, -20.3019) (58.6825, -20.3969) knots 0 0 0 0 0.321396 0.321396 0.48066 0.48066 0.635294 0.635294 1 1 1 1
  line L72 (58.6825, -20.3969) -> (58.6795, -20.4078)
  arc A36 (57.7229, -20.4199) -> (58.6795, -20.4078) centre (58.1994, -20.2682) ccw
  line L73 (57.7229, -20.4199) -> (57.7196, -20.4091)
  spline S64 degree 3 poles (57.7196, -20.4091) (57.7009, -20.3486) (57.6772, -20.2869) (57.6237, -20.1841) (57.5939, -20.1379) (57.5341, -20.0751) (57.5073, -20.0533) (57.4376, -20.0163) (57.4042, -20.0116) (57.3328, -20.0052) (57.267, -20.006) (57.2495, -20.0054) knots 0 0 0 0 0.221578 0.221578 0.405224 0.405224 0.524808 0.524808 0.681199 0.681199 1 1 1 1
  spline S65 degree 3 poles (57.2495, -20.0054) (57.1985, -20.0033) (57.1469, -19.9951) (57.0712, -20.0021) (57.0385, -20.0083) (56.9635, -20.0481) (56.931, -20.076) (56.8364, -20.1797) (56.7854, -20.2788) (56.7488, -20.3705) knots 0 0 0 0 0.321396 0.321396 0.48066 0.48066 0.635294 0.635294 1 1 1 1
  line L74 (56.7488, -20.3705) -> (56.7446, -20.381)
  arc A37 (55.792, -20.293) -> (56.7446, -20.381) centre (56.2817, -20.1919) ccw
  line L75 (55.792, -20.293) -> (55.7899, -20.2819)
  spline S66 degree 3 poles (55.7899, -20.2819) (55.7775, -20.2198) (55.7604, -20.156) (55.718, -20.0482) (55.6931, -19.9991) (55.6403, -19.9304) (55.616, -19.9059) (55.5505, -19.8618) (55.5178, -19.8537) (55.4474, -19.8398) (55.3819, -19.8338) (55.3645, -19.8313) knots 0 0 0 0 0.221578 0.221578 0.405224 0.405224 0.524808 0.524808 0.681199 0.681199 1 1 1 1
  spline S67 degree 3 poles (55.3645, -19.8313) (55.314, -19.8239) (55.2636, -19.8104) (55.1875, -19.8094) (55.1544, -19.8121) (55.0757, -19.8439) (55.0404, -19.8682) (54.9355, -19.9615) (54.8744, -20.0548) (54.8284, -20.1421) knots 0 0 0 0 0.321396 0.321396 0.48066 0.48066 0.635294 0.635294 1 1 1 1
  line L76 (54.8284, -20.1421) -> (54.8231, -20.1521)
  arc A38 (53.885, -19.965) -> (54.8231, -20.1521) centre (54.3826, -19.9157) ccw
  line L77 (53.885, -19.965) -> (53.884, -19.9538)
  spline S68 degree 3 poles (53.884, -19.9538) (53.8782, -19.8903) (53.8677, -19.8245) (53.8365, -19.7126) (53.8169, -19.6615) (53.7715, -19.5879) (53.7499, -19.5611) (53.6983, -19.5181) (53.6752, -19.507) (53.6593, -19.5007) knots 0 0 0 0 0.348162 0.348162 0.633559 0.633559 0.819801 0.819801 1 1 1 1
  line L78 (53.6593, -19.5007) -> (53.3721, -19.4256)
  spline S69 degree 3 poles (53.3721, -19.4256) (53.3465, -19.4215) (53.3255, -19.4211) (53.2835, -19.4253) (53.2619, -19.4305) (53.1991, -19.4532) (53.1601, -19.4776) (53.0549, -19.5618) (52.9925, -19.6393) (52.9424, -19.7142) knots 0 0 0 0 0.112636 0.112636 0.2383 0.2383 0.490329 0.490329 1 1 1 1
  line L79 (52.9424, -19.7142) -> (52.9361, -19.7236)
  arc A39 (52.0227, -19.4395) -> (52.9361, -19.7236) centre (52.5227, -19.4424) ccw
  ellipse E4 centre (51.3276, -20.1713) end of major axis (50.8167, -21.3897) minor radius 0.5115 (52.0227, -19.4395) -> (51.9479, -19.0534) ccw
  line L80 (51.9479, -19.0534) -> (51.3324, -18.8925)
  ellipse E5 centre (51.1696, -19.8639) end of major axis (50.7829, -20.8737) minor radius 0.4341 (51.3324, -18.8925) -> (51.1114, -19.0915) ccw
  line L81 (51.1114, -19.0915) -> (51.1042, -19.1002)
  arc A40 (50.2255, -18.7222) -> (51.1042, -19.1002) centre (50.7224, -18.7774) ccw
  line L82 (50.2255, -18.7222) -> (50.2269, -18.711)
  ellipse E6 centre (49.9179, -18.9244) end of major axis (49.7181, -19.5766) minor radius 0.2583 (50.2269, -18.711) -> (50.2349, -18.6056) ccw
  line L83 (50.2349, -18.6056) -> (49.2657, -18.3523)
  arc A41 (48.5635, -18.1688) -> (49.2657, -18.3523) centre (49.0016, -17.9278) ccw
  line L84 (48.5635, -18.1688) -> (0.6482, -5.6452)
  arc A42 (0.6482, -5.6452) -> (0.6565, -5.8882) centre (1.1884, -5.7484) ccw
  arc A43 (0.5152, -6.0882) -> (0.6565, -5.8882) centre (0.5017, -5.9288) ccw
  arc A44 (0.0559, -6.1097) -> (0.5152, -6.0882) centre (0, 0) ccw
  arc A45 (-0.1034, -5.9237) -> (0.0559, -6.1097) centre (0.0545, -5.9498) ccw
  arc A46 (-0.1034, -5.9237) -> (-0.3185, -5.3925) centre (-0.6461, -5.8343) ccw
  line L85 (-0.3185, -5.3925) -> (-0.7156, -5.2887)
  arc A47 (-0.7156, -5.2887) -> (-1.1952, -5.8028) centre (-0.6461, -5.8343) ccw
  arc A48 (-1.3914, -5.9495) -> (-1.1952, -5.8028) centre (-1.3549, -5.7937) ccw
  arc A49 (-1.8348, -5.828) -> (-1.3914, -5.9495) centre (0, 0) ccw
  arc A50 (-1.9289, -5.6019) -> (-1.8348, -5.828) centre (-1.7868, -5.6754) ccw
  arc A51 (-1.9289, -5.6019) -> (-2.0498, -4.94) centre (-2.4174, -5.3491) ccw
  line L86 (-2.0498, -4.94) -> (-2.5378, -4.8125)
  arc A52 (-2.5378, -4.8125) -> (-2.9299, -5.1495) centre (-2.4174, -5.3491) ccw
  arc A53 (-3.1617, -5.2283) -> (-2.9299, -5.1495) centre (-3.079, -5.0914) ccw
  arc A54 (-3.546, -4.9758) -> (-3.1617, -5.2283) centre (0, 0) ccw
  arc A55 (-3.5655, -4.7316) -> (-3.546, -4.9758) centre (-3.4531, -4.8455) ccw
  arc A56 (-3.5655, -4.7316) -> (-4.3777, -3.9921) centre (-3.952, -4.3403) ccw
  arc A57 (-4.6226, -3.9954) -> (-4.3777, -3.9921) centre (-4.5016, -3.8908) ccw
  arc A58 (-4.91, -3.6365) -> (-4.6226, -3.9954) centre (0, 0) ccw
  arc A59 (-4.8532, -3.3982) -> (-4.91, -3.6365) centre (-4.7814, -3.5412) ccw
  arc A60 (-4.8532, -3.3982) -> (-5.3971, -2.4439) centre (-5.0998, -2.9066) ccw
  arc A61 (-5.631, -2.3714) -> (-5.3971, -2.4439) centre (-5.4836, -2.3093) ccw
  arc A62 (-5.7934, -1.9412) -> (-5.631, -2.3714) centre (0, 0) ccw
  arc A63 (-5.6658, -1.7322) -> (-5.7934, -1.9412) centre (-5.6417, -1.8904) ccw
  arc A64 (-5.6658, -1.7322) -> (-5.8882, -0.6565) centre (-5.7484, -1.1884) ccw
  arc A65 (-6.0882, -0.5152) -> (-5.8882, -0.6565) centre (-5.9288, -0.5017) ccw
  arc A66 (-6.1097, -0.0559) -> (-6.0882, -0.5152) centre (0, 0) ccw
  arc A67 (-5.9237, 0.1034) -> (-6.1097, -0.0559) centre (-5.9498, -0.0545) ccw
  arc A68 (-5.9237, 0.1034) -> (-5.8028, 1.1952) centre (-5.8343, 0.6461) ccw
  arc A69 (-5.9495, 1.3914) -> (-5.8028, 1.1952) centre (-5.7937, 1.3549) ccw
  arc A70 (-5.828, 1.8348) -> (-5.9495, 1.3914) centre (0, 0) ccw
  arc A71 (-5.6019, 1.9289) -> (-5.828, 1.8348) centre (-5.6754, 1.7868) ccw
  arc A72 (-5.6019, 1.9289) -> (-5.1495, 2.9299) centre (-5.3491, 2.4174) ccw
  arc A73 (-5.2283, 3.1617) -> (-5.1495, 2.9299) centre (-5.0914, 3.079) ccw
  arc A74 (-4.9758, 3.546) -> (-5.2283, 3.1617) centre (0, 0) ccw
  arc A75 (-4.7316, 3.5655) -> (-4.9758, 3.546) centre (-4.8455, 3.4531) ccw
  arc A76 (-4.7316, 3.5655) -> (-3.9921, 4.3777) centre (-4.3403, 3.952) ccw
  arc A77 (-3.9954, 4.6226) -> (-3.9921, 4.3777) centre (-3.8908, 4.5016) ccw
  arc A78 (-3.6365, 4.91) -> (-3.9954, 4.6226) centre (0, 0) ccw
  arc A79 (-3.3982, 4.8532) -> (-3.6365, 4.91) centre (-3.5412, 4.7814) ccw
  arc A80 (-3.3982, 4.8532) -> (-2.4439, 5.3971) centre (-2.9066, 5.0998) ccw
  arc A81 (-2.3714, 5.631) -> (-2.4439, 5.3971) centre (-2.3093, 5.4836) ccw
  arc A82 (-1.9412, 5.7934) -> (-2.3714, 5.631) centre (0, 0) ccw
  arc A83 (-1.7322, 5.6658) -> (-1.9412, 5.7934) centre (-1.8904, 5.6417) ccw
  arc A84 (-1.7322, 5.6658) -> (-0.6565, 5.8882) centre (-1.1884, 5.7484) ccw
  arc A85 (-0.5152, 6.0882) -> (-0.6565, 5.8882) centre (-0.5017, 5.9288) ccw
  arc A86 (-0.0559, 6.1097) -> (-0.5152, 6.0882) centre (0, 0) ccw
  arc A87 (0.1034, 5.9237) -> (-0.0559, 6.1097) centre (-0.0545, 5.9498) ccw
  arc A88 (0.1034, 5.9237) -> (0.2618, 5.4408) centre (0.6461, 5.8343) ccw
  line L87 (0.2618, 5.4408) -> (1.1484, 5.6104)
  arc A89 (1.1484, 5.6104) -> (1.1952, 5.8028) centre (0.6461, 5.8343) ccw
  arc A90 (1.3914, 5.9495) -> (1.1952, 5.8028) centre (1.3549, 5.7937) ccw
  arc A91 (1.8348, 5.828) -> (1.3914, 5.9495) centre (0, 0) ccw
  arc A92 (1.9235, 5.7586) -> (1.8348, 5.828) centre (1.7868, 5.6754) ccw
  line L88 (52.1516, -24.1871) -> (-2.5827, -9.8813)
  arc A93 (-1.9181, 10.0315) -> (-2.5827, -9.8813) centre (0, 0) ccw
  line L89 (-1.9181, 10.0315) -> (53.6482, 20.6561)
  arc A94 (52.1516, -24.1871) -> (53.6482, 20.6561) centre (57.9677, -1.9346) ccw
  line L90 (21.175, 21.125) -> (-21.175, 21.125)
  line L91 (-21.175, 21.125) -> (-21.175, -21.125)
  line L92 (-21.175, -21.125) -> (21.175, -21.125)
  line L93 (21.175, -21.125) -> (21.175, 21.125)
  circle A95 centre (0, 0) radius 12.1
  circle A96 centre (15.4774, -15.5226) radius 1.3645
  circle A97 centre (-15.4774, 15.5226) radius 1.3645
  circle A98 centre (15.5226, 15.4774) radius 1.3645
  circle A99 centre (-15.5226, -15.4774) radius 1.3645
  point P0 (0, 0)
  point P1 (21.175, -16.0908)
  point P2 (16.7025, -14.9218)
  point P3 (14.7029, -14.3992)
  point P4 (3.695, -11.522)
  point P5 (4.455, 11.25)
  point P6 (21.175, 14.447)
  dimension "d3" = 3
  constraints: 4 end point, 4 point on circle, 2 centre point, 10 other
  measures "d3" distance between parallel lines of L0 L88
extrude "Extrusion2" add sketch "Sketch2" along normal blind 17 contours A95 L88 A96 L93 L92 L91 L90 L89
fillet "Fillet1" radius 30 2 edges at (3.695, -11.522, 16) (4.455, 11.25, 16)
fillet "Fillet2" radius 1 2 edges at (16.7025, -14.9218, 16) (14.7029, -14.3992, 16)
sketch "Sketch4" plane through (0, 0, 24.5) normal (0, 0, 1) x (1, 0, 0)
  circle A0 centre (15.4774, -15.5226) radius 3.1 projected
  arc A1 (14.1427, -15.2387) -> (13.4175, -14.0632) centre (13.1646, -15.0307) ccw projected
  line L0 (13.4175, -14.0632) -> (9.4746, -13.0327) projected
  arc A2 (9.4746, -13.0327) -> (0.5427, -12.0878) centre (1.8884, -42.0576) ccw projected
  arc A3 (1.3475, 12.0247) -> (0.5427, -12.0878) centre (0, 0) ccw projected
  arc A4 (1.3475, 12.0247) -> (10.3225, 12.3719) centre (4.6883, 41.8381) ccw projected
  line L1 (10.3225, 12.3719) -> (21.175, 14.447) projected
  line L2 (21.175, 14.447) -> (21.175, 21.125) projected
  line L3 (21.175, 21.125) -> (-21.175, 21.125) projected
  line L4 (-21.175, 21.125) -> (-21.175, -21.125) projected
  line L5 (-21.175, -21.125) -> (21.175, -21.125) projected
  line L6 (21.175, -21.125) -> (21.175, -16.0908) projected
  line L7 (21.175, -16.0908) -> (17.9879, -15.2578) projected
  arc A5 (17.9879, -15.2578) -> (16.7802, -15.9281) centre (17.735, -16.2253) ccw projected
  arc A6 (14.1427, -15.2387) -> (16.7802, -15.9281) centre (15.4774, -15.5226) ccw projected
  circle A7 centre (-15.4774, 15.5226) radius 1.3645 projected
  circle A8 centre (-15.5226, -15.4774) radius 1.3645 projected
  circle A9 centre (15.5226, 15.4774) radius 1.3645 projected
  line L8 (-12.4226, -15.4774) -> (-12.4226, -21.125) projected
  arc A10 (-12.4226, -15.4774) -> (-15.5226, -12.3774) centre (-15.5226, -15.4774) ccw projected
  line L9 (-21.175, -12.3774) -> (-15.5226, -12.3774) projected
  point P0 (0, 0)
  point P1 (12.83, -13.9097)
  point P2 (18.5754, -15.4113)
extrude "Extrusion5" cut sketch "Sketch4" against normal blind 4 contours A0 L0 A1 A6 A5 L7 | L5 L4 L9 A10 L8 picked at (16.0692, -17.9552)
sketch "Sketch5" plane through (0, 0, 24.5) normal (0, 0, 1) x (1, 0, 0)
  circle A0 centre (-0.0226, -15.5) radius 1.8 projected
  point P0 (0, 0)
hole "Hole1" at (-0.0226, -15.5, 24.5) direction (0, 0, -1) diameter 4.2 depth 6 counterbore diameter 5 counterbore depth 0.6
sketch "Sketch6" plane through (0, 0, 24.5) normal (0, 0, 1) x (1, 0, 0)
  arc A0 (1.3475, 12.0247) -> (0.5427, -12.0878) centre (0, 0) ccw projected
  line L0 (-12.1, 0) -> (-12.1, -21.125)
  line L1 (-21.175, -21.125) -> (21.175, -21.125) projected
  arc A1 (-10.8027, -21.5756) -> (-12.1, -21.125) centre (-12.1, -23.218) ccw
  line L2 (-10.8027, -21.5756) -> (22.2759, -25.092)
  line L3 (22.2759, -25.092) -> (22.6931, 1.6092)
  line L4 (22.6931, 1.6092) -> (-12.1, 0)
  point P0 (0, 0)
  constraints: 8 end point, 3 point on circle, 2 point on line, 1 centre point, 1 vertical
extrude "Extrusion6" cut sketch "Sketch6" against normal up to surface (17 mm away)
sketch "Sketch7" plane through (0, 0, 24.5) normal (0, 0, 1) x (1, 0, 0)
  line L0 (-21.175, -21.125) -> (-21.175, -12.3774) projected
  line L1 (-21.175, -12.3774) -> (-3.1739, -12.3774)
  line L2 (-3.1739, -12.3774) -> (-3.1739, -27.2229)
  line L3 (-3.1739, -27.2229) -> (-4.8462, -27.2299)
  line L4 (-4.8462, -27.2299) -> (-21.8521, -26.4093)
  line L5 (-21.8521, -26.4093) -> (-21.175, -12.3774)
  point P0 (0, 0)
  constraints: 10 end point, 2 perpendicular, 1 horizontal
extrude "Extrusion7" cut sketch "Sketch7" against normal blind 10
move faces "Move1" translate (0, 0, 7.5) faces at (-16.3207, -19.694, 14.5)
move faces "Move2" translate (0, 0, -2) faces at (-16.3207, -19.694, 22)
move faces "Move3" translate (0, 0, -3) faces at (-16.3207, -19.694, 20)
sketch "Sketch8" plane through (0, 0, 24.5) normal (0, 0, 1) x (1, 0, 0)
  circle A0 centre (15.5226, 15.4774) radius 1.3645 projected
  arc A1 (1.3475, 12.0247) -> (-12.1, 0) centre (0, 0) ccw projected
  arc A2 (1.3475, 12.0247) -> (10.3225, 12.3719) centre (4.6883, 41.8381) ccw projected
  line L0 (10.3225, 12.3719) -> (21.175, 14.447) projected
  line L1 (21.175, 14.447) -> (21.175, 21.125) projected
  line L2 (21.175, 21.125) -> (-21.175, 21.125) projected
  line L3 (-21.175, 21.125) -> (-21.175, -12.3774) projected
  circle A3 centre (-15.4774, 15.5226) radius 1.3645 projected
  circle A4 centre (15.5226, 15.4774) radius 1.3645 projected
  line L4 (20.175, 15.2739) -> (10.1347, 13.3541)
  arc A5 (1.4588, 13.0185) -> (10.1347, 13.3541) centre (4.6883, 41.8381) ccw
  arc A6 (1.4588, 13.0185) -> (-13.0003, 1.613) centre (0, 0) ccw
  line L5 (-13.0003, 1.613) -> (-20.175, 1.613)
  line L6 (-20.175, 1.613) -> (-20.175, 20.125)
  line L7 (-20.175, 20.125) -> (20.175, 20.125)
  line L8 (20.175, 20.125) -> (20.175, 15.2739)
  line L9 (20.175, 15.2739) -> (21.175, 15.4651)
  line L10 (21.175, -21.125) -> (21.175, 21.125) projected
  line L11 (10.1347, 13.3541) -> (5.2624, 12.4225)
  line L12 (5.2624, 12.4225) -> (-1.1831, 11.1901)
  line L13 (-21.175, -12.3774) -> (-12.1, -12.3774) projected
  line L14 (-12.1, -12.3774) -> (-12.1, 0) projected
  point P0 (0, 0)
  point P1 (2.5902, 11.9116)
  point P2 (16.5515, 14.5811)
  point P3 (14.897, 14.2647)
  dimension "d37" = 1
  constraints: 16 end point, 4 point on circle, 3 point on line, 2 centre point, 1 tangent, 4 other
  measures "d37" distance between parallel lines of L0 L4
extrude "Extrusion8" cut sketch "Sketch8" against normal up to surface (17 mm away) contours A0 L4 L9 L1 L0 A2 L12 L11
fillet "Fillet3" radius 1 2 edges at (16.5515, 14.5811, 16) (14.897, 14.2647, 16)
move faces "Move4" translate (0, 0, -3) faces at (4.9007, -19.6319, 0)
move faces "Move5" translate (0, 0, -3) faces at (-16.3207, -19.694, 17)
chamfer "Chamfer2" distance 10.5 angle 60 1 edges at (-16.6375, -12.3774, 24.5) measured on face at (-16.6375, -12.3774, 24)
sketch "Sketch9" plane through (0, 0, 24.5) normal (0, 0, 1) x (1, 0, 0)
  line L0 (110.8694, -1.8119) -> (-349.1301, -1.1403) projected
  line L1 (-10.6143, 5.8092) -> (-21.175, 5.8092) projected
  arc A0 (1.3475, 12.0247) -> (-10.6143, 5.8092) centre (0, 0) ccw projected
  arc A1 (1.3475, 12.0247) -> (2.5902, 11.9116) centre (4.6883, 41.8381) ccw projected
  line L2 (2.5902, 11.9116) -> (13.4029, 13.9791) projected
  arc A2 (13.4029, 13.9791) -> (14.191, 15.1795) centre (13.2151, 14.9613) ccw projected
  arc A3 (16.8702, 15.6918) -> (14.191, 15.1795) centre (15.5226, 15.4774) ccw projected
  arc A4 (16.8702, 15.6918) -> (18.0455, 14.8668) centre (17.8577, 15.849) ccw projected
  line L3 (18.0455, 14.8668) -> (21.175, 15.4651) projected
  line L4 (21.175, 15.4651) -> (21.175, 21.125) projected
  line L5 (21.175, 21.125) -> (-21.175, 21.125) projected
  line L6 (-21.175, 21.125) -> (-21.175, 5.8092) projected
  circle A5 centre (-15.4774, 15.5226) radius 1.3645 projected
  arc A6 (-10.6143, 5.8092) -> (-12.1, 0) centre (0, 0) ccw projected
  line L7 (-10.6143, 5.8092) -> (-21.175, 5.8092) projected
  line L8 (-21.175, 5.8092) -> (-21.175, -12.3774) projected
  line L9 (-21.175, -12.3774) -> (-12.1, -12.3774) projected
  line L10 (-12.1, -12.3774) -> (-12.1, 0) projected
  line L11 (21.175, -1.6809) -> (21.175, 15.4651)
  arc A7 (14.191, 15.1795) -> (16.8702, 15.6918) centre (15.5226, 15.4774) ccw projected
  point P0 (0, 0)
  point P1 (-21.175, -1.6191)
  constraints: 2 end point, 1 parallel, 1 point on line
ref_plane "Work Plane2" through (32.1178, -1.5407, 70) normal (0, 0, 1) x (1, 0, 0)
extrude "Extrusion9" add sketch "Sketch9" along normal up to surface (45.5 mm away) contours L0 L10 A6 A0 A1 L2 A2 A7 A4 L3 L11 | L0 L8 L1 A6 L10 | L3 A4 A3 A2 L2 A1 A0 L1 L6 L5 L4
sketch "Sketch10" plane through (-21.175, 21.125, 70) normal (0, 0, 1) x (1, 0, 0)
  circle A0 centre (36.6976, -5.6476) radius 1.3645 projected
  circle A1 centre (36.6976, -5.6476) radius 3
  circle A2 centre (5.6976, -5.6024) radius 1.3645 projected
  circle A3 centre (5.6976, -5.6024) radius 3
  point P0 (21.175, -21.125)
  dimension "d52" = 6
  dimension "d53" = 6
  constraints: 2 centre point, 2 coincident
  measures "d52" diameter of A1
  measures "d53" diameter of A3
extrude "Extrusion10" cut sketch "Sketch10" against normal blind 26
sketch "Sketch11" plane through (-21.175, 21.125, -3) normal (0, 1, 0) x (1, 0, 0)
  circle A0 centre (78.3331, -62.9998) radius 1.7 projected
  circle A1 centre (78.3331, -43) radius 1.7 projected
  line L0 (33.6976, -73) -> (33.6976, -47) projected
  line L1 (39.6976, -73) -> (39.6976, -47) projected
  line L2 (8.6976, -73) -> (8.6976, -47) projected
  line L3 (2.6976, -73) -> (2.6976, -47) projected
  point P0 (21.175, -3)
  point P1 (29.6976, -62.9998)
  point P2 (12.6976, -62.9998)
  point P3 (29.6976, -43)
  point P4 (33.6976, -60)
  point P5 (8.6976, -60)
  point P6 (12.6976, -43)
  dimension "d56" = 17
  dimension "d57" = 4
  dimension "d58" = 4
  dimension "d59" = 0
  constraints: 3 horizontal alignment, 2 midpoint
  measures "d56" distance of point (12.698, -63) point (29.698, -63)
  measures "d57" horizontal distance of point (33.698, -60) point (29.698, -63)
  measures "d58" horizontal distance of point (8.698, -60) point (12.698, -63)
  measures "d59" horizontal distance of point (29.698, -43) point (29.698, -63)
hole "Hole2" at (8.5226, 21.125, 59.9998) at (-8.4774, 21.125, 59.9998) at (8.5226, 21.125, 40) at (-8.4774, 21.125, 40) direction (0, -1, 0) diameter 3.4 end through all counterbore diameter 6.5 counterbore depth 3.4 clearance for "Socket Head Cap Screw ISO 4762" size "M3" standard "ISO"
move faces "Move6" translate (0, 1.5, 0) faces at (8.9175, 17.725, 62.6852) (8.7841, 19.9917, 63.2392) (10.1912, 4.7984, 60.3252) (-8.0825, 17.725, 62.6852) (-8.2159, 19.9917, 63.2392) (-6.8088, 4.815, 60.3252) (8.9175, 17.725, 42.6854) (8.7841, 19.9917, 43.2395) (10.1912, 4.7984, 40.3255)
sketch "Sketch12" plane through (-21.175, -21.125, -3) normal (-1, 0, 0) x (0, 0, 1)
  line L0 (27.5, 19.4441) -> (73, 19.4441) projected
  line L1 (17, 0) -> (17, 8.7476) projected
  line L2 (27.5, 19.4441) -> (17, 8.7476)
  line L3 (27.5, 26.9342) -> (17, 8.7476) projected
  line L4 (27.5, 26.9342) -> (27.5, 19.5059) projected
  line L5 (27.5, 19.5059) -> (73, 19.5059) projected
  line L6 (73, 19.5059) -> (73, 42.25) projected
  line L7 (0, 42.25) -> (73, 42.25) projected
  line L8 (0, 42.25) -> (0, 0) projected
  line L9 (0, 0) -> (17, 0) projected
  line L10 (17, 0) -> (17, 8.7476) projected
  line L11 (27.5, 19.5059) -> (17, 8.7476)
  point P0 (3, 21.125)
  constraints: 4 end point
extrude "Extrusion11" add sketch "Sketch12" against normal up to surface (9.075 mm away) contours L3 L4 L11
delete faces "Delete Face2" heal yes whole lump no faces at (-11.3821, 5.1944, 24.1451)
move faces "Move7" translate (0, 0.312, 0) faces at (8.9175, 19.225, 62.6852) (9.0439, 20.4917, 63.2077) (10.1912, 4.7984, 60.3252) (8.6594, 18.725, 61.6943) (-8.0825, 19.225, 62.6852) (-7.9561, 20.4917, 63.2077) (-6.8088, 4.815, 60.3252) (-8.3406, 18.725, 61.6943) (-8.0825, 17.725, 42.6854) (-7.9561, 20.4917, 43.2079) (-8.2159, 18.725, 43.2395) (-6.8088, 4.815, 40.3255) (8.9175, 19.225, 42.6854) (9.0439, 20.4917, 43.2079) (10.1912, 4.7984, 40.3255) (8.6594, 18.725, 41.6945)
move faces "Move8" translate (0, 1.5, 0) faces at (-8.0825, 18.037, 42.6854) (-8.2159, 20.5957, 43.2395) (-8.2159, 19.433, 43.2395) (-7.9561, 18.829, 43.2079) (-6.8088, 4.815, 40.3255) (-8.2047, 17.829, 41.678)
move faces "Move9" translate (0, 0, -0.4) faces at (3.9253, 2.8661, 24.5)
body "Solid1"
